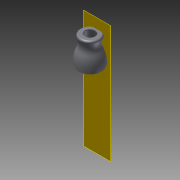
# Autodesk Inventor part: New
Saved by Autodesk Inventor 2011 SP2 (Build 150309200, 309)
## iProperties
Created: 2012-04-18
Part Number: New
Document SubType Name: Modeling
Designer: sungwook
Density: 8.08 g/cm^3
Material: Stainless Steel
Mass: 44.6509 g
Surface Area: 48.11 cm^2
Volume: 5.5261 cm^3
Author: sungwook
Autodesk Inventor part; units mm, degrees
ref_plane "YZ Plane" through (0, 0, 0) normal (1, 0, 0) x (0, 1, 0)
ref_plane "XY Plane" through (0, 0, 0) normal (0, 0, 1) x (1, 0, 0)
sketch "Block1" plane through (0, 0, 0) normal (0, 0, 1) x (1, 0, 0)
  line L0 (-13, 33) -> (0, 33)
  line L1 (0, 33) -> (0, 31.984)
  line L2 (0, 0) -> (-7.5, 0)
  line L3 (-5.5, 31.984) -> (0, 31.984)
  spline S0 degree 4 poles (-5.5, 31.984) (-8.3018, 31.984) (-14.9701, 28.615) (-2.778, 19.5085) (-12.1324, 9.4997) (-13.0429, 3.8555) (-13.0429, 0) knots 0 0 0 0 0 0.349618 0.599618 1 1 1 1 1
  spline S1 degree 4 poles (-5.5, 33) (-8.695, 33) (-16.2444, 29.0645) (-3.8371, 19.8287) (-13.0244, 9.853) (-14.2875, 3.9571) (-14.2875, 0) knots 0 0 0 0 0 0.356198 0.606198 1 1 1 1 1
  line L4 (-13.0429, 0) -> (13.0429, 0)
  line L5 (13.0429, 0) -> (13.0429, -90)
  line L6 (13.0429, -90) -> (-13.0429, -90)
  line L7 (-13.0429, -90) -> (-13.0429, 0)
  line L8 (0, 33) -> (0, 31.984)
  line L9 (0, 0) -> (14.2875, 0)
  line L10 (14.2875, 0) -> (14.2875, -90)
  line L11 (14.2875, -90) -> (-14.2875, -90)
  line L12 (-14.2875, -90) -> (-14.2875, 0)
  line L13 (-14.2875, 0) -> (-13.0429, 0)
  line L14 (-13.0429, 0) -> (-12.0269, 0)
  line L15 (-12.0269, 0) -> (-12.0269, -5)
  line L16 (-12.0269, -5) -> (-13.0429, -5)
  line L17 (-13.0429, -5) -> (-13.0429, 0)
  spline S2 degree 4 poles (-12.0269, 0) (-12.0269, 1.8651) (-12.9196, 3.9842) (-12.4898, 5.3301) (-12.0051, 6.8202) knots 0 0 0 0 0 1 1 1 1 1
  point P0 (-5.8286, -1.9888)
  point P1 (-2.75, 31.984)
  point P2 (-10.8475, 28.6822)
  point P3 (-8.5755, 20.4298)
  point P4 (-10.7949, 9.9764)
  point P5 (-11.8109, 29.0047)
  point P6 (-9.5915, 20.5086)
  point P7 (-11.8109, 10.2944)
  point P8 (-12.757, 3.7934)
  point P9 (-12.2202, 6.1237)
  point P10 (-12.4905, 4.0174)
  dimension "d0" = 1.016
  dimension "d1" = 1.016
  dimension "d2" = 1.016
  dimension "d3" = 1.016
  dimension "d4" = 90
  dimension "d5" = 26.0858
  dimension "d6" = 33
  dimension "d7" = 5.5
  dimension "d8" = 28.575
  dimension "d9" = 5
  dimension "d10" = 1.016
  measures "d0" distance between parallel lines of L3 L0
  measures "d1" distance of point (-10.847, 28.682) point (-11.811, 29.005)
  measures "d2" horizontal distance of point (-10.795, 9.976) point (-11.811, 10.294)
  measures "d3" horizontal distance of point (-8.576, 20.43) point (-9.592, 20.509)
  measures "d4" distance of L6.end L4.start
  measures "d5" distance of L4.end L4.start
  measures "d6" distance between parallel lines of L2 L0
  measures "d7" distance of L0.end point (-5.5, 33)
  measures "d8" distance of L9.end L12.end
  measures "d9" distance of L15.end L14.end
  measures "d10" distance between parallel lines of L15 L7
sketch "Sketch2" plane through (0, 0, 0) normal (1, 0, 0) x (0, 1, 0)
  point P0 (0, 0)
sketch "Sketch3" plane through (0, 0, 0) normal (1, 0, 0) x (0, 1, 0)
  line L0 (0, -114.856) -> (0, 59.1357) projected
  line L1 (0, 29) -> (-11.8121, 29)
  line L2 (-13.0429, 0) -> (-12.0429, 0)
  line L3 (-12.0429, 0) -> (-12.0429, -3)
  line L4 (-12.0429, -3) -> (-13.0429, -3)
  line L5 (-13.0429, -3) -> (-13.0429, 0)
  line L6 (-14.2875, 0) -> (-14.2875, -7.5209)
  spline S0 degree 4 poles (-8.7178, 15.3035) (-9.5873, 11.2411) (-11.424, 6.9381) (-12.0429, 3.6863) (-12.0429, 0) knots 0 0 0 0 0 1 1 1 1 1
  spline S1 degree 4 poles (-11.8121, 29) (-11.4923, 26.2408) (-6.533, 15.3028) (-13.5295, 15.4591) (-14.2875, 3.7094) (-14.2875, 0) knots 0 0 0 0 0 0.596386 1 1 1 1 1
  line L7 (-14.2875, 0) -> (-13.0429, 0)
  line L8 (0, 29) -> (-11.625, 29)
  line L9 (-11.625, 28) -> (0, 28)
  line L10 (0, 28) -> (0, 29)
  line L11 (-6, 28) -> (-8.7178, 15.3035)
  point P0 (0, 0)
  point P1 (-12.0269, 0)
  point P2 (-6, 29)
  point P3 (-11.1126, 6.8247)
  point P4 (-10.2731, 22.7051)
  point P5 (-10.2729, 16.6704)
  point P6 (-12.5423, 11.3252)
  dimension "d12" = 29
  dimension "d13" = 14.2875
  dimension "d14" = 3
  dimension "d15" = 1
  dimension "d17" = 13.0429
  dimension "d18" = 1
  dimension "d35" = 6
  constraints: 22 end point, 4 parallel, 3 point on line, 2 horizontal, 2 perpendicular, 2 vertical, 11 other
  measures "d12" distance of point (0, 0) L1.start
  measures "d13" distance of point (0, 0) L6.start
  measures "d14" distance from line of L3.end L2
  measures "d15" distance between parallel lines of L3 L5
  measures "d17" distance of point (0, 0) L2.start
  measures "d18" distance between parallel lines of L9 L8
  measures "d35" distance of L11.start L9.end
revolve "Revolution1" add sketch "Sketch3" angle 360 about axis through (0, 0, -10) along (0, 0, 1)
fillet "Fillet1" radius 2 1 edges at (0, 11.8121, 29)
fillet "Fillet2" [suppressed]
hole "Hole1" at (0, 0, 29) direction (0, 0, -1) diameter 12 end through all
ref_plane "Work Plane2" through (0, 8.3, 0) normal (0, 1, 0) x (-1, 0, 0)
sketch "Sketch6" plane through (0, 8.3, 0) normal (0, 1, 0) x (-1, 0, 0)
  arc A0 (2.6663, 15.3035) -> (-2.6663, 15.3035) centre (-2.6663, 15.3035) ccw projected
  arc A1 (-2.6663, 15.3035) -> (-8.7259, 0) centre (-8.7259, 0) ccw projected
  line L0 (-8.7259, 0) -> (-8.7259, -3) projected
  line L1 (-8.7259, -3) -> (-10.0612, -3) projected
  line L2 (-10.0612, -3) -> (-10.0612, 0) projected
  line L3 (-10.0612, 0) -> (-11.6294, 0) projected
  arc A2 (-11.6294, 0) -> (-7.5554, 26.4676) centre (-7.5554, 26.4676) ccw projected
  arc A3 (-7.5554, 26.4676) -> (-4.1863, 29) centre (-4.1863, 29) ccw projected
  line L4 (-4.1863, 29) -> (4.1863, 29) projected
  arc A4 (4.1863, 29) -> (7.5554, 26.4676) centre (7.5554, 26.4676) ccw projected
  arc A5 (7.5554, 26.4676) -> (11.6294, 0) centre (11.6294, 0) ccw projected
  line L5 (11.6294, 0) -> (10.0612, 0) projected
  line L6 (10.0612, 0) -> (10.0612, -3) projected
  line L7 (10.0612, -3) -> (8.7259, -3) projected
  line L8 (8.7259, -3) -> (8.7259, 0) projected
  arc A6 (8.7259, 0) -> (2.6663, 15.3035) centre (2.6663, 15.3035) ccw projected
  line L9 (12.0429, -3) -> (-12.0429, -3) projected
  line L10 (0, -114.856) -> (0, 59.1357) projected
  line L11 (-10, 8) -> (10, 8)
  line L12 (10, 8) -> (10, -3)
  line L13 (10, -3) -> (-10, -3)
  line L14 (-10, -3) -> (-10, 8)
  point P0 (0, 0)
  point P1 (0, 8)
  dimension "d46" = 11
  dimension "d47" = 20
  constraints: 8 end point, 2 parallel, 1 horizontal, 1 horizontal alignment, 1 midpoint, 1 perpendicular, 1 point on line, 1 vertical alignment, 6 other
  measures "d46" distance of L12.end L11.end
  measures "d47" distance of L11.end L11.start
extrude "Extrusion1" cut sketch "Sketch6" along normal through all contours L11 L12 A2 L10 | L10 A2 L0 A1 L14 L11 | L10 L9 L0 A2 | A2 L12 A6 L8 L9 L10 | A2 A1 L0 | L0 L1 L14 A1 A2 | A2 A1 L14 | L8 A6 L12 L7
equation "\"d0\" = d11"
equation "\"d1\" = d11"
equation "\"d2\" = d11"
equation "\"d3\" = d11"
equation "\"d11\" = 1.016"
body "Solid1"
